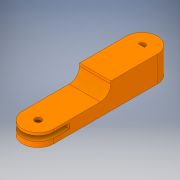
# Autodesk Inventor part: ArmThicker
Saved by Autodesk Inventor 2017 (Build 210142000, 142)
## iProperties
Created: 2017-03-25
Part Number: ArmThicker
Material: Generic
Document SubType Name: Modeling
Designer: Parshant Bombhi
Density: 1 g/cm^3
Appearance: Default
LengthOfArm_Thicker: 6.500 in
Thickness_Thicker: 1.250 in
Author: Parshant Bombhi
Autodesk Inventor part; units mm, degrees
ref_plane "YZ Plane" through (0, 0, 0) normal (1, 0, 0) x (0, 1, 0)
ref_plane "XZ Plane" through (0, 0, 0) normal (0, 1, 0) x (-1, 0, 0)
ref_plane "XY Plane" through (0, 0, 0) normal (0, 0, 1) x (1, 0, 0)
sketch "Sketch1" plane through (0, 0, 0) normal (0, 1, 0) x (-1, 0, 0)
  line L0 (0, -19.05) -> (0, -146.05)
  line L1 (19.05, -165.1) -> (19.05, -165.1)
  line L2 (38.1, -146.05) -> (38.1, -19.05)
  line L3 (19.05, 0) -> (19.05, 0)
  arc A0 (0, -146.05) -> (19.05, -165.1) centre (19.05, -146.05) ccw
  arc A1 (19.05, -165.1) -> (38.1, -146.05) centre (19.05, -146.05) ccw
  arc A2 (38.1, -19.05) -> (19.05, 0) centre (19.05, -19.05) ccw
  arc A3 (19.05, 0) -> (0, -19.05) centre (19.05, -19.05) ccw
  circle A4 centre (19.05, -19.05) radius 3.9688
  circle A5 centre (19.05, -146.05) radius 3.9688
  point P0 (0, 0)
  point P1 (0, -165.1)
  point P2 (38.1, -165.1)
  dimension "d0" = 38.1
  dimension "LengthOfArm_Thicker" = 165.1
  dimension "d2" = 19.05
  dimension "d3" = 7.9375
  dimension "Motor_Shaft_Diameter" = 7.9375
  constraints: 8 end point, 8 point on circle, 8 tangent, 6 centre point, 6 point on line, 3 equal radius, 3 perpendicular, 2 coincident, 1 vertical
  measures "d0" distance of point (0, -165.1) point (38.1, -165.1)
  measures "LengthOfArm_Thicker" distance of point (0, 0) point (0, -165.1)
  measures "d2" radius of A0
  measures "d3" diameter of A4
  measures "Motor_Shaft_Diameter" diameter of A5
extrude "Extrusion1" add sketch "Sketch1" along normal blind 31.75
sketch "Sketch3" plane through (0, 0, -19.05) normal (1, 0, 0) x (0, 0, -1)
  line L0 (-57.15, 6.35) -> (19.05, 6.35)
  line L1 (19.05, 6.35) -> (19.05, 12.7)
  line L2 (19.05, 12.7) -> (-57.15, 12.7)
  line L3 (-57.15, 12.7) -> (-57.15, 6.35)
  line L4 (-19.05, 0) -> (-19.05, 31.75) projected
  line L5 (-57.15, 6.35) -> (19.05, 12.7) construction
  line L6 (19.05, 6.35) -> (-57.15, 12.7) construction
  line L7 (0, 0) -> (-19.05, 0) projected
  line L8 (-19.05, 0) -> (-19.05, 31.75) projected
  line L9 (-19.05, 15.875) -> (69.85, 15.875)
  line L10 (69.85, 15.875) -> (69.85, 31.75)
  line L11 (127, 31.75) -> (0, 31.75) projected
  line L12 (0, 31.75) -> (-19.05, 31.75) projected
  line L13 (69.85, 31.75) -> (-19.05, 31.75)
  line L14 (-19.05, 0) -> (-19.05, 31.75) projected
  line L15 (-19.05, 31.75) -> (-19.05, 15.875)
  point P0 (-19.05, 9.525)
  point P1 (-19.05, 9.525)
  dimension "d15" = 6.35
  dimension "d19" = 6.35
  dimension "d20" = 15.875
  dimension "d21" = 88.9
  constraints: 20 end point, 4 perpendicular, 3 midpoint, 2 parallel, 2 point on line, 1 collinear, 1 horizontal
  measures "d15" distance of L0.end L1.end
  measures "d19" distance between parallel lines of L7 L0
  measures "d20" distance between parallel lines of L12 L9
  measures "d21" distance between parallel lines of L10 L4
extrude "Extrusion3" cut sketch "Sketch3" against normal up to next
fillet "Fillet3" radius 12.7 1 edges at (-19.05, 15.875, -88.9)
sketch "Sketch4" plane through (0, 31.75, 0) normal (0, 1, 0) x (1, 0, 0)
  circle A0 centre (-19.05, 146.05) radius 3.9687 projected
  line L0 (-9.6345, 145.2562) -> (-28.4655, 145.2562)
  line L1 (-28.4655, 145.2562) -> (-28.4655, 138.9062)
  line L2 (-28.4655, 138.9062) -> (-9.6345, 138.9062)
  line L3 (-9.6345, 138.9062) -> (-9.6345, 145.2562)
  line L4 (-9.6345, 145.2562) -> (-28.4655, 138.9062) construction
  line L5 (-28.4655, 145.2562) -> (-9.6345, 138.9062) construction
  point P0 (0, 0)
  point P1 (-19.05, 142.0812)
  dimension "d23" = 6.35
  constraints: 12 end point, 2 midpoint, 2 parallel, 1 horizontal, 1 perpendicular, 1 vertical alignment, 1 other
  measures "d23" distance of L0.end L1.end
extrude "Extrusion4" add sketch "Sketch4" against normal up to surface (31.75 mm away) contours L0 A0 | A0 L0 L3 L2 L1 picked at (-18.2787, 143.8235)
equation "\"Thickness_Thicker\" = 2 * Thickness_Thiner"
equation "\"Thickness_Thiner\" = 15.875"
body "Solid1"
